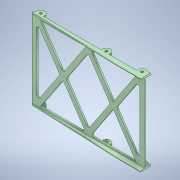
# Autodesk Inventor part: BodyStructure Plate
Saved by Autodesk Inventor 2022.2 (Build 262287030, 287C)
## iProperties
Created: 2019-11-07
Part Number: BodyStructure Plate
Material: solidworks materials|ABS
Document SubType Name: Modeling
Designer: Jochen
Density: 1.02 g/cm^3
Appearance: 151,157,178
Sending System: SolidWorks 2017
Last Author: Felix
Last Saved: 2021-02-23
Author: Jochen
Autodesk Inventor part; units mm, degrees
ref_plane "YZ Plane" through (0, 0, 0) normal (1, 0, 0) x (0, 1, 0)
ref_plane "XZ Plane" through (0, 0, 0) normal (0, 1, 0) x (-1, 0, 0)
ref_plane "Work Plane1" through (0, 0, 30) normal (0, 0, 1) x (1, 0, 0)
sketch "Sketch1" plane through (0, 0, 30) normal (0, 0, 1) x (1, 0, 0)
  line L0 (-26, -45.5) -> (26, -45.5)
  line L1 (26, 45.5) -> (-26, 45.5)
  line L2 (26, 42) -> (26, 42)
  line L3 (0, -63.7) -> (0, 63.7) construction
  line L4 (-125.2, 0) -> (51.2, 0) construction
  line L5 (-8.7421, -3.6057) -> (-34.3232, -42)
  line L6 (-37, -37) -> (-12.3479, 0)
  line L7 (-37, 37) -> (-12.3479, 0)
  line L8 (-8.7421, 3.6057) -> (-34.3232, 42)
  line L9 (26, -37) -> (26, -37)
  line L10 (26, -45.5) -> (26, -37)
  line L11 (26, 42) -> (26, 45.5)
  line L12 (26, -37) -> (26, 42)
  line L13 (21, -39.2276) -> (21, 39.2276)
  line L14 (21, -39.2276) -> (-5.1364, 0)
  line L15 (-5.1364, 0) -> (21, 39.2276)
  line L16 (-26, 45.5) -> (-100, 45.5)
  line L17 (-100, 45.5) -> (-100, -45.5)
  line L18 (-100, -45.5) -> (-26, -45.5)
  line L19 (-65.2579, 3.6057) -> (-39.6768, 42)
  line L20 (-65.2579, -3.6057) -> (-39.6768, -42)
  line L21 (-37, -37) -> (-61.6521, 0)
  line L22 (-37, 37) -> (-61.6521, 0)
  line L23 (-95, 39.2276) -> (-68.8636, 0)
  line L24 (-95, -39.2276) -> (-68.8636, 0)
  line L25 (-95, 39.2276) -> (-95, -39.2276)
  line L26 (-37, -45.5) -> (-37, 45.5) construction
  arc A0 (-39.6768, 42) -> (-34.3232, 42) centre (-37, 40.2165) ccw construction
  line L27 (-65.2579, -45.5) -> (-65.2579, 45.5) construction
  circle A1 centre (-65.2579, 0) radius 3.6057 construction
  line L28 (-65.2579, 3.6057) -> (-90.839, 42)
  line L29 (-65.2579, -3.6057) -> (-90.839, -42)
  line L30 (-39.6768, 42) -> (-90.839, 42)
  line L31 (-39.6768, -42) -> (-90.839, -42)
  line L32 (-90.839, 42) -> (-95, 42) construction
  line L33 (-95, 42) -> (-95, 39.2276) construction
  arc A2 (-95, 39.2276) -> (-90.839, 42) centre (-92.9195, 40.6138) ccw construction
  line L34 (16.839, 42) -> (-8.7421, 3.6057)
  line L35 (-8.7421, 42) -> (-8.7421, -42) construction
  line L36 (-8.7421, -3.6057) -> (16.839, -42)
  line L37 (16.839, -42) -> (-34.3232, -42)
  line L38 (-34.3232, 42) -> (16.839, 42)
  point P0 (0, 0)
  point P1 (0, 3.7162)
  point P2 (-52.4673, 22.8029)
  dimension "d7" = 91
  dimension "d136" = 5
  dimension "d138" = 5
  dimension "d149" = 126
  dimension "d150" = 26
  dimension "d152" = 63
  dimension "d153" = 5
  dimension "d156" = 3.5
  constraints: 75 end point, 13 point on line, 11 parallel, 8 horizontal, 8 point on circle, 7 perpendicular, 4 midpoint, 4 tangent, 3 centre point, 3 collinear, 3 vertical, 2 equal length, 8 other
  measures "d7" distance between parallel lines of L1 L0
  measures "d136" distance between parallel lines of L13 L12
  measures "d138" distance between parallel lines of L17 L25
  measures "d149" distance between parallel lines of L17 L12
  measures "d150" distance from line of L3 L1.start
  measures "d152" distance between parallel lines of L26 L12
  measures "d153" distance between parallel lines of L22 L19
  measures "d156" distance between parallel lines of L1 L38
extrude "Extrusion1" add sketch "Sketch1" along normal blind 13
fillet "Fillet1" radius 2 15 edges at (-34.3232, -42, 36.5) (-12.3479, 0, 36.5) (-34.3232, 42, 36.5) (-5.1364, 0, 36.5) (21, -39.2276, 36.5) (-37, 37, 36.5) (21, 39.2276, 36.5) (-65.2579, -3.6057, 36.5) (-95, 39.2276, 36.5) (-61.6521, 0, 36.5) (-65.2579, 3.6057, 36.5) (-68.8636, 0, 36.5) (-39.6768, -42, 36.5) (-95, -39.2276, 36.5) (-37, -37, 36.5)
sketch "Sketch3" plane through (0, 0, 0) normal (1, 0, 0) x (0, 1, 0)
  line L0 (0, -8.6) -> (0, 51.6) construction
  line L1 (-70.794, 0) -> (70.7157, 0) construction
  line L2 (-45.5, 43) -> (45.5, 43) construction
  line L3 (45.5, 43) -> (-45.5, 43) construction
  line L4 (45.5, 30) -> (-45.5, 30) construction
  line L5 (-45.5, 30) -> (45.5, 30) construction
  line L6 (45.5, 30) -> (45.5, 43) construction
  line L7 (45.5, 30) -> (45.5, 43) construction
  line L8 (37, 30) -> (37, 42.5) construction
  line L9 (37, 30) -> (37, 42.5) construction
  line L10 (-45.5, 30) -> (-45.5, 43) construction
  line L11 (-45.5, 30) -> (-45.5, 43) construction
  line L12 (-37, 30) -> (-37, 41) construction
  line L13 (-45.5, 30) -> (-45.5, 38.5)
  line L14 (-45.5, 43) -> (-45, 43)
  line L15 (-45, 43) -> (-43.5441, 39)
  line L16 (-43.5441, 39) -> (43.5441, 39)
  line L17 (45.5, 40.0648) -> (45.5, 30)
  line L18 (-45.25, 43) -> (-45.25, 30) construction
  line L19 (-45.5, 43) -> (-45.5, 38.5)
  line L20 (-43.5, 30) -> (-43.5, 37.5)
  line L21 (-43.5, 37.5) -> (-42, 37.5)
  line L22 (40.5, 30) -> (40.5, 43) projected
  line L23 (45.5, 40.0648) -> (45.5, 43)
  line L24 (45.5, 43) -> (45, 43)
  line L25 (45.5, 43) -> (-45.5, 43) projected
  line L26 (45, 43) -> (43.5441, 39)
  line L27 (43.5, 37.5) -> (43.5, 30)
  line L28 (32.0296, 37.5) -> (43.5, 37.5)
  line L29 (-42, 37.5) -> (32.0296, 37.5)
  line L30 (-45.5783, 30) -> (-43.5, 30)
  line L31 (45.5, 30) -> (-45.5, 30) projected
  point P0 (0, 0)
  point P1 (37, 41)
  point P2 (37, 41)
  point P3 (37, 41)
  point P4 (-37, 30)
  point P5 (1.0399, 30)
  point P6 (37, 30)
  point P7 (-37, 30)
  point P8 (-45.5, 34.25)
  point P9 (-1.0399, 30)
  point P10 (21.2913, 30)
  point P11 (20.2514, 30)
  point P12 (-20.2514, 30)
  point P13 (-21.2913, 30)
  dimension "d29" = 0.5
  dimension "d85" = 2
  dimension "d88" = 7.5
  dimension "d89" = 20
  dimension "d90" = 1.5
  constraints: 34 end point, 3 collinear, 2 horizontal, 2 midpoint, 2 perpendicular, 2 point on line, 1 parallel, 1 vertical, 8 other
  measures "d29" distance of L3.end L14.end
  measures "d85" distance between parallel lines of L20 L10
  measures "d88" distance of L20.start L20.end
  measures "d89" angle of L15 L10
  measures "d90" distance between parallel lines of L16 L29
extrude "Extrusion3" cut sketch "Sketch3" along normal through all both and the other way through all contours L13 L19 L14 L15 L16 L22 L28 L29 L21 L20 L30 | L22 L16 L26 L24 L23 L17 L31 L27 L28 keep common part
sketch "Sketch11" plane through (0, 0, 0) normal (0, 1, 0) x (-1, 0, 0)
  line L0 (100, 43) -> (-26, 43) construction
  line L1 (0.1527, 42.9379) -> (27.014, 41.8785)
  line L2 (6, 30) -> (26, 30)
  arc A0 (0.1527, 42.9379) -> (-3, 43) centre (-3, -37) ccw
  line L3 (-26, 30) -> (100, 30) construction
  line L4 (-26, 43) -> (-26, 39) projected
  line L5 (27.014, 41.8785) -> (100, 39)
  line L6 (-3, 43) -> (-26, 43)
  line L7 (-26, 43) -> (-26, 30)
  line L8 (-26, 30) -> (6, 30)
  line L9 (100, 30) -> (-26, 30) projected
  line L10 (100, 37.5) -> (95, 37.5) projected
  line L11 (95, 39) -> (100, 39) projected
  line L12 (12.7511, 37.5) -> (4.7331, 37.5) projected
  line L13 (4.7331, 37.5) -> (4.7331, 39) projected
  line L14 (4.7331, 39) -> (12.7511, 39) projected
  line L15 (-21, 37.5) -> (-26, 37.5) projected
  line L16 (-26, 37.5) -> (-26, 39) projected
  line L17 (-26, 39) -> (-21, 39) projected
  line L18 (-21, 39) -> (-21, 37.5) projected
  line L19 (100, 39) -> (100, 37.5) projected
  line L20 (95, 37.5) -> (95, 39) projected
  line L21 (69.2669, 37.5) -> (61.2489, 37.5) projected
  line L22 (61.2489, 37.5) -> (61.2489, 39) projected
  line L23 (61.2489, 39) -> (69.2669, 39) projected
  line L24 (69.2669, 39) -> (69.2669, 37.5) projected
  line L25 (12.7511, 39) -> (12.7511, 37.5) projected
  line L26 (100, 30) -> (100, 43) projected
  line L27 (100, 39) -> (100, 30)
  line L28 (100, 30) -> (26, 30)
  point P0 (0, 0)
  point P1 (-26, 39)
  point P2 (99, 39)
  point P3 (-26, 39)
  point P4 (99, 39)
  dimension "d91" = 80
  dimension "d94" = 4
  dimension "d95" = 23
  constraints: 16 end point, 3 collinear, 2 point on circle, 2 point on line, 2 tangent, 1 centre point, 1 perpendicular, 1 vertical
  measures "d91" radius of A0
  measures "d94" distance from line of L5.end L0
  measures "d95" distance from line of L6.start L4
extrude "Extrusion11" cut sketch "Sketch11" along normal through all both and the other way through all contours L1 L5 L11 L20 L10 L26 L9 L2 L8 L7 L15 L18 L17 L4 L6 A0 | L19 L10 L20 L11 | L17 L18 L15 L7 | L12 L13 L14 L25 | L21 L22 L23 L24 keep common part
sketch "Sketch12" plane through (0, 0, 0) normal (0, 1, 0) x (-1, 0, 0)
  circle A0 centre (-20, 35.5) radius 1.5
  circle A1 centre (-20, 35.5) radius 3
  circle A2 centre (20, 35.5) radius 1.5
  circle A3 centre (20, 35.5) radius 3
  line L0 (-26, 37.5) -> (-26, 30) construction
  line L1 (-20, 35.5) -> (20, 35.5) construction
  arc A4 (22.8284, 32) -> (24.5, 35.5) centre (20, 35.5) ccw
  arc A5 (15.5, 35.5) -> (22.8284, 32) centre (20, 35.5) ccw
  line L2 (15.5, 37) -> (-15.5, 37)
  arc A6 (-22.8284, 32) -> (-15.5, 35.5) centre (-20, 35.5) ccw
  line L3 (24.5, 35.5) -> (24.5, 36)
  arc A7 (22.8284, 32) -> (22.8284, 32) centre (19.5074, 36.1096) ccw
  line L4 (-26, 32) -> (-22.8284, 32)
  line L5 (-26, 43) -> (-26, 32)
  line L6 (-26, 43) -> (26, 43)
  line L7 (100, 39) -> (-26, 39) projected
  line L8 (-22.8284, 39) -> (22.9247, 39)
  arc A8 (-24.5, 35.5) -> (-22.8284, 32) centre (-20, 35.5) ccw
  line L9 (15.5, 35.5) -> (15.5, 37)
  line L10 (24.5, 36) -> (24.5, 37.5)
  line L11 (24.5, 37.5) -> (22.2361, 37.5)
  line L12 (-24.5, 37) -> (-24.5, 35.5)
  line L13 (-15.5, 37) -> (-15.5, 35.5)
  line L14 (-26, 37.5) -> (100, 37.5) projected
  line L15 (-22.2361, 37.5) -> (-24.5, 37.5)
  line L16 (-24.5, 37) -> (-24.5, 37.5)
  line L17 (-17.7639, 37.5) -> (-15.5, 37.5)
  line L18 (-18.6348, 37.5) -> (-1.7039, 37.5) projected
  line L19 (-15.5, 37) -> (-15.5, 36.8517)
  line L20 (-15.5, 37) -> (-15.5, 37.5)
  line L21 (15.5, 37) -> (15.5, 37.5)
  line L22 (16.9309, 37.5) -> (-16.9309, 37.5) projected
  line L23 (15.5, 37.5) -> (17.7639, 37.5)
  line L24 (8.7421, 37.5) -> (32.2518, 37.5) projected
  circle A9 centre (94, 35.5) radius 1.5
  circle A10 centre (94, 35.5) radius 3
  arc A11 (89.5, 35.5) -> (98.5, 35.5) centre (94, 35.5) ccw
  line L25 (100, 37.5) -> (100, 30) projected
  line L26 (24.5, 37) -> (89.5, 37)
  line L27 (89.5, 37) -> (89.5, 35.5)
  line L28 (93.3278, 37.5) -> (62.783, 37.5) projected
  line L29 (89.5, 37.5) -> (91.7639, 37.5)
  line L30 (100, 37.5) -> (-26, 37.5) projected
  line L31 (96.2361, 37.5) -> (98.5, 37.5)
  line L32 (98.5, 35.5) -> (98.5, 37.5)
  line L33 (100, 37.5) -> (100, 43)
  line L34 (100, 43) -> (26, 43)
  line L35 (89.5, 37) -> (89.5, 37.5)
  point P0 (0, 0)
  point P1 (-24.4142, 32)
  point P2 (22.8284, 32)
  point P3 (17.4019, 37)
  point P4 (-17.4019, 37)
  point P5 (-22.5981, 37)
  point P6 (1.7039, 37.5)
  point P7 (18.6348, 37.5)
  point P8 (59, 39)
  point P9 (24.5, 37.5)
  point P10 (-26, 37.5)
  point P11 (98.5, 37.5)
  point P12 (89.5, 37.5)
  point P13 (24.5, 37)
  dimension "d98" = 3
  dimension "d99" = 6
  dimension "d100" = 6
  dimension "d102" = 7.5
  dimension "d110" = 4.5
  dimension "d113" = 6
  dimension "d114" = 11
  dimension "d141" = 6
  dimension "d151" = 40
  constraints: 54 end point, 21 point on circle, 15 point on line, 12 centre point, 9 vertical, 8 coincident, 8 equal radius, 7 tangent, 4 horizontal, 2 collinear, 2 perpendicular, 1 midpoint, 10 other
  measures "d98" diameter of A0
  measures "d99" diameter of A1
  measures "d100" distance from line of L1.start L0
  measures "d102" vertical distance of L5.start A0.centre
  measures "d110" radius of A4
  measures "d113" distance between parallel lines of L6 L2
  measures "d114" distance between parallel lines of L6 L4
  measures "d141" distance from line of L25 A9.centre
  measures "d151" distance of A2.centre A0.centre
extrude "Extrusion12" cut sketch "Sketch12" along normal through all both and the other way through all contours A0 | A2 | A9
extrude "Extrusion13" cut sketch "Sketch12" along normal through all both and the other way through all contours A0 | A1 L14 | A1 L14 L20 L13 A6 A8 L12 L16 | L14 A1 | A1 L14 L5 L7 A7 | L16 L12 A8 L4 L5 L14 | L14 A7 L2 L20 | L5 L6 L34 L33 L7 A7 | A7 L14 L21 L2 | A7 L7 L14 L11 A3 | L21 L14 A3 L11 L10 L3 A4 A5 L9 | A7 L7 | L7 L33 L14 A10 A7 | L26 L10 L14 A7 | A7 L14 L35 L26 | L14 A3 | A3 L14 | L35 L14 A10 L32 A11 L27 | A10 L14 | L14 A10 | A2 | A9 keep common part
extrude "Extrusion14" add sketch "Sketch12" along normal blind 1 from surface at -43.5 contours A1 L14 | A1 L14 L20 L13 A6 A8 L12 L16 | L14 A1 | L21 L14 A3 L11 L10 L3 A4 A5 L9 | L14 A3 | A3 L14 | L35 L14 A10 L32 A11 L27 | A10 L14 | L14 A10
extrude "Extrusion15" add sketch "Sketch12" against normal blind 1 from surface at 43.5 contours A1 L14 | A1 L14 L20 L13 A6 A8 L12 L16 | L14 A1 | L21 L14 A3 L11 L10 L3 A4 A5 L9 | L14 A3 | A3 L14 | L35 L14 A10 L32 A11 L27 | L14 A10 picked at (94.5816, 37.3297)
chamfer "Chamfer2" distance 1 distance2 2 1 edges at (20, -42.5, 31) measured on face at (20, -43, 31)
chamfer "Chamfer3" distance 1 distance2 2 1 edges at (20, 42.5, 31) measured on face at (20, 43, 31)
chamfer "Chamfer4" distance 2 distance2 1 2 edges at (-20, 42.5, 31) (-24.5, 42.5, 36.5) measured on face at (-20, 42.5, 31.5) measured on face at (-24, 42.5, 36.5)
chamfer "Chamfer5" distance 2 distance2 1 3 edges at (-20, -42.5, 31) (-15.5, -42.5, 36.5) (-24.5, -42.5, 36.5) measured on face at (-24, -42.5, 36.5) measured on face at (-16, -42.5, 36.5) measured on face at (-20, -42.5, 31.5)
chamfer "Chamfer6" distance 2 distance2 1 3 edges at (-94, -42.5, 31) (-89.5, -42.5, 36.5) (-98.5, -42.5, 36.5) measured on face at (-90, -42.5, 36.5) measured on face at (-98, -42.5, 36.5) measured on face at (-94, -42.5, 31.5)
chamfer "Chamfer7" distance 2 distance2 1 3 edges at (-94, 42.5, 31) (-98.5, 42.5, 36.5) (-89.5, 42.5, 36.5) measured on face at (-94, 42.5, 31.5) measured on face at (-90, 42.5, 36.5) measured on face at (-98, 42.5, 36.5)
body "Solid1"
body "Solid2"
